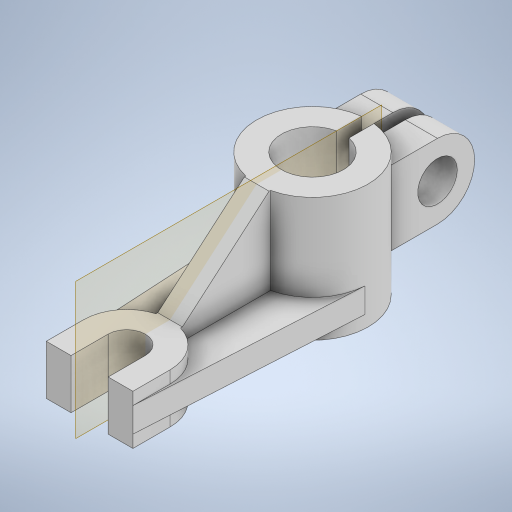
# Autodesk Inventor part: 2
Saved by Autodesk Inventor 2023 (Build 270158000, 158)
## iProperties
Created: 2023-09-26
Part Number: 2
Material: Všeobecné
Document SubType Name: Modeling
Designer: clu40164
Mass: 106.922 g
Surface Area: 280.787 cm^2
Volume: 106.922 cm^3
Density: 1 g/cm^3
Appearance: Výchozí
Author: clu40164
Autodesk Inventor part; units mm, degrees
ref_plane "YZ Plane" through (0, 0, 0) normal (1, 0, 0) x (0, 1, 0)
ref_plane "XZ Plane" through (0, 0, 0) normal (0, 1, 0) x (-1, 0, 0)
ref_plane "XY Plane" through (0, 0, 0) normal (0, 0, 1) x (1, 0, 0)
sketch "Náčrt3" plane through (0, 0, 0) normal (0, 1, 0) x (-1, 0, 0)
  line L0 (18.7116, 64.0709) -> (8.7116, 64.0709)
  line L1 (8.7116, 64.0709) -> (8.7116, 49.0709)
  arc A0 (-6.2884, 49.0709) -> (8.7116, 49.0709) centre (1.2116, 49.0709) ccw
  line L2 (-6.2884, 49.0709) -> (-6.2884, 64.0709)
  line L3 (-6.2884, 64.0709) -> (-16.2884, 64.0709)
  arc A1 (3.6769, -38.1765) -> (-1.3231, -38.1765) centre (1.1769, -25.9291) ccw
  arc A2 (3.6769, -48.2898) -> (-1.3231, -48.2898) centre (1.1769, -25.9291) ccw
  line L4 (18.7116, 64.0709) -> (23.6423, -24.681)
  line L5 (-16.2884, 64.0709) -> (-21.2875, -24.6635)
  arc A3 (-16.2884, 49.0709) -> (18.7116, 49.0709) centre (1.2116, 49.0709) ccw
  line L6 (18.7116, 49.0709) -> (18.7116, 64.0709)
  line L7 (-16.2884, 49.0709) -> (-16.2884, 64.0709)
  line L8 (-1.3231, -38.1765) -> (-1.3231, -48.2898)
  line L9 (3.6769, -48.2898) -> (3.6769, -38.1765)
  point P0 (0, 0)
  dimension "d0" = 10
  dimension "d1" = 10
  dimension "d2" = 15
  dimension "d3" = 15
  dimension "d4" = 7.5
  dimension "d5" = 25
  dimension "d6" = 45
  dimension "d7" = 75
  dimension "d11" = 3.18
  dimension "d12" = 22.2368
  dimension "d13" = 18.7116
  dimension "d16" = 15.0347
  dimension "d17" = 20.0347
  constraints: 20 end point, 10 point on circle, 6 tangent, 4 centre point, 4 vertical, 2 coincident, 2 parallel, 1 perpendicular
  measures "d0" distance of L0.start L0.end
  measures "d1" distance of L2.end L3.end
  measures "d2" distance of L0.end L1.end
  measures "d3" distance of L2.start L2.end
  measures "d4" radius of A0
  measures "d5" diameter of A1
  measures "d6" diameter of A2
  measures "d7" distance of A1.centre A0.centre
  measures "d11" angle of L4 L6
  measures "d12" distance from line of point (0, 0) L4
  measures "d13" distance from line of point (0, 0) L6
  measures "d16" distance between parallel lines of L9 L6
  measures "d17" distance between parallel lines of L8 L6
extrude "Vysunutí1" add sketch "Náčrt3" against normal blind 5 contours L6 A3 L7 L3 L2 A0 L1 L0 | A2 L9 A1 L8
extrude "Vysunutí2" add sketch "Náčrt3" along normal blind 10 contours L4 A2 L5 L7 A3 L6
extrude "Vysunutí3" add sketch "Náčrt3" along normal blind 15 contours L6 A3 L7 L3 L2 A0 L1 L0
extrude "Vysunutí4" add sketch "Náčrt3" along normal blind 45 contours A2 L9 A1 L8
ref_plane "Pracovní rovina1" through (-1.3339, 0, 376.8696) normal (1, 0, 0.0004) x (0, 1, 0)
sketch "Náčrt4" plane through (-1.3339, 0, 376.8696) normal (1, 0, 0.0004) x (0, 1, 0)
  line L0 (45, -425.1604) -> (45, -380.2987) projected
  line L1 (15, -345.2987) -> (45, -380.2987)
  line L2 (45, -380.2987) -> (45, -385.2987)
  line L3 (45, -385.2987) -> (10, -385.2987)
  line L4 (10, -401.5419) -> (10, -312.7919) projected
  line L5 (15, -345.2987) -> (15, -327.7919) projected
  line L6 (10, -345.2987) -> (10, -385.2987)
  line L7 (15, -345.2987) -> (15, -343.2987)
  line L8 (15, -343.2987) -> (10, -343.2987)
  line L9 (10, -327.7919) -> (10, -345.2987) projected
  line L10 (15, -343.2987) -> (10, -343.2987)
  line L11 (10, -345.2987) -> (10, -343.2987)
  point P0 (0, -376.8701)
  point P1 (45, -425.1584)
  point P2 (15, -327.8055)
  point P3 (10, -327.8055)
  dimension "d26" = 5
  dimension "d28" = 42
  constraints: 16 end point, 4 point on line, 3 perpendicular, 2 collinear
  measures "d26" distance of L0.end L2.end
  measures "d28" distance between parallel lines of L10 L3
extrude "Vysunutí5" add sketch "Náčrt4" along normal blind 5
extrude "Vysunutí6" add sketch "Náčrt4" against normal blind 5
sketch "Náčrt7" plane through (-3.6769, -5, -38.1765) normal (1, 0, 0) x (0, 0, -1)
  line L0 (0, 15) -> (10.2526, 15)
  line L1 (10.2526, 15) -> (22.7526, 15)
  line L2 (22.7526, 45) -> (0, 45)
  line L3 (0, 45) -> (0, 15)
  arc A0 (22.7526, 15) -> (22.7526, 45) centre (22.7526, 30) ccw
  circle A1 centre (22.7526, 30) radius 8
  point P0 (-38.1765, 5)
  dimension "d45" = 12.5
  dimension "d46" = 30
  dimension "d47" = 16
  dimension "d48" = 10
  dimension "d49" = 38.1765
  dimension "d50" = 22.7525
  constraints: 8 end point, 2 centre point, 2 point on circle, 2 tangent, 1 coincident, 1 horizontal, 1 parallel, 1 perpendicular, 1 point on line
  measures "d45" distance of L0.end L1.end
  measures "d46" distance of L1.end L2.start
  measures "d47" diameter of A1
  measures "d48" distance from line of point (-38.177, 5) L0
  measures "d49" distance from line of point (-38.177, 5) L3
  measures "d50" distance from line of L2.start L3
extrude "Vysunutí7" add sketch "Náčrt7" along normal blind 18
extrude "Vysunutí8" cut sketch "Náčrt7" along normal blind 5
extrude "Vysunutí9" add sketch "Náčrt7" against normal blind 13
